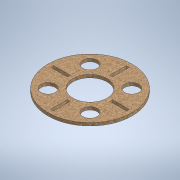
# Autodesk Inventor part: Anillo de Centrado
Saved by Autodesk Inventor 2020 (Build 240168000, 168)
## iProperties
Created: 2021-09-30
Part Number: Anillo de Centrado
Material: MDF Medium Density Fiberboard
Document SubType Name: Modeling
Designer: Carlos
Density: 0.8 g/cm^3
Appearance: Cardboard - Corrugated
Mass: 5.3112 g
Surface Area: 67.9447 cm^2
Volume: 6.63899 cm^3
Author: Carlos
Autodesk Inventor part; units mm, degrees
ref_plane "YZ Plane" through (0, 0, 0) normal (1, 0, 0) x (0, 1, 0)
ref_plane "XZ Plane" through (0, 0, 0) normal (0, 1, 0) x (-1, 0, 0)
ref_plane "XY Plane" through (0, 0, 0) normal (0, 0, 1) x (1, 0, 0)
sketch "Sketch1" plane through (0, 0, 0) normal (0, 1, 0) x (-1, 0, 0)
  circle A0 centre (0, 0) radius 35.17
  circle A1 centre (0, 0) radius 14.25
  line L0 (14.25, 0) -> (35.17, 0)
  line L1 (-17.4726, 17.4726) -> (36, -36)
  line L2 (0, 0) -> (50.9117, 0) construction
  line L3 (0, 0) -> (0, -35.17)
  line L4 (0, -35.17) -> (0, -14.25)
  circle A2 centre (0, 0) radius 24.71
  circle A3 centre (17.4726, -17.4726) radius 6
  line L5 (17.4726, 17.4726) -> (-36, -36)
  circle A4 centre (-17.4726, -17.4726) radius 6
  circle A5 centre (17.4726, 17.4726) radius 6
  circle A6 centre (-17.4726, 17.4726) radius 6
  point P0 (0, -24.71)
  dimension "d0" = 70.34
  dimension "d1" = 28.5
  dimension "d2" = 45
  dimension "d20" = 12
  dimension "d21" = 12
  dimension "d22" = 12
  dimension "d23" = 12
  constraints: 12 end point, 9 point on circle, 7 centre point, 6 coincident, 5 point on line, 2 horizontal, 1 midpoint, 1 symmetric about line, 1 vertical
  measures "d0" diameter of A0
  measures "d1" diameter of A1
  measures "d2" angle of L1 L2
  measures "d20" diameter of A3
  measures "d21" diameter of A4
  measures "d22" diameter of A5
  measures "d23" diameter of A6
extrude "Extrusion1" add sketch "Sketch1" along normal blind 2.5 contours L0 A2 A5 A6 A4 L5 A0 | A0 L1 A3 A2 L0 | L5 A4 A2 L3 A0 | A0 L3 A2 A3 L1 | A2 A3 L1 A1 L0 | L0 A1 L5 A5 A2 | A2 A4 L5 A1 L3 | L3 A1 L1 A3 A2 | A2 A6 L1 A1 L5 A4 | A1 L1 A6 A2 A5 L5
sketch "Sketch2" plane through (0, 2.5, 0) normal (0, 1, 0) x (1, 0, 0)
  circle A0 centre (0, 0) radius 35.17 projected
  circle A1 centre (0, 0) radius 14.25 projected
  line L0 (-14.25, 0) -> (-35.17, 0)
  line L1 (-24.71, 0) -> (-24.71, 1.25)
  line L2 (-24.71, 1.25) -> (-24.71, -1.25)
  line L3 (-24.71, 1.25) -> (-31.71, 1.25)
  line L4 (-24.71, 1.25) -> (-17.71, 1.25)
  line L5 (-17.71, 1.25) -> (-17.71, -1.25)
  line L6 (-17.71, -1.25) -> (-31.71, -1.25)
  line L7 (-31.71, -1.25) -> (-31.71, 1.25)
  line L8 (-1.25, -24.71) -> (-1.25, -17.71)
  line L9 (-1.25, -17.71) -> (1.25, -17.71)
  line L10 (1.25, -17.71) -> (1.25, -31.71)
  line L11 (1.25, -31.71) -> (-1.25, -31.71)
  line L12 (-1.25, -24.71) -> (-1.25, -31.71)
  line L13 (24.71, -1.25) -> (17.71, -1.25)
  line L14 (17.71, -1.25) -> (17.71, 1.25)
  line L15 (17.71, 1.25) -> (31.71, 1.25)
  line L16 (31.71, 1.25) -> (31.71, -1.25)
  line L17 (24.71, -1.25) -> (31.71, -1.25)
  line L18 (1.25, 24.71) -> (1.25, 17.71)
  line L19 (1.25, 17.71) -> (-1.25, 17.71)
  line L20 (-1.25, 17.71) -> (-1.25, 31.71)
  line L21 (-1.25, 31.71) -> (1.25, 31.71)
  line L22 (1.25, 24.71) -> (1.25, 31.71)
  dimension "d24" = 1.25
  dimension "d25" = 2.5
  dimension "d26" = 7
  dimension "d27" = 7
  dimension "d30" = 360
  constraints: 46 end point, 4 perpendicular, 2 horizontal, 2 horizontal alignment, 1 midpoint, 1 point on line, 1 vertical, 43 other
  measures "d24" distance of L1.start L1.end
  measures "d25" distance of L1.end L2.end
  measures "d26" distance of L1.end L3.end
  measures "d27" distance of L1.end L4.end
extrude "Extrusion2" cut sketch "Sketch2" against normal blind 22.25 contours L7 L3 L1 L0 | L0 L2 L6 L7 | L1 L4 L5 L0 | L0 L5 L6 L2 | L8 L9 L10 L11 L12 | L13 L14 L15 L16 L17 | L18 L19 L20 L21 L22
pattern_circular "Circular Pattern1" count 4 over 360 about axis through (0, -10, 0) along (0, 1, 0) of "Extrusion2"
body "Solid1"
